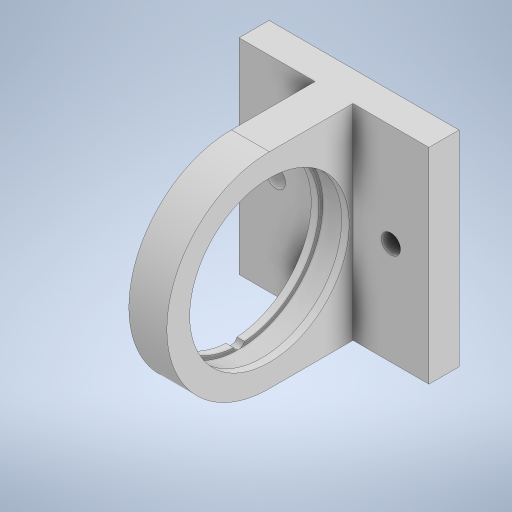
# Autodesk Inventor part: antenna_rad_outter
Saved by Autodesk Inventor 2024 (Build 280153000, 153)
## iProperties
Created: 2025-12-27
Part Number: antenna_rad_outter
Material: Generic
Document SubType Name: Modeling
Designer: schar
Density: 1 g/cm^3
Appearance: Default
Author: schar
Autodesk Inventor part; units mm, degrees
ref_plane "YZ Plane" through (0, 0, 0) normal (1, 0, 0) x (0, 1, 0)
ref_plane "XZ Plane" through (0, 0, 0) normal (0, 1, 0) x (-1, 0, 0)
sketch "Sketch15" plane through (0, 0, 0) normal (1, 0, 0) x (0, 1, 0)
  circle A0 centre (0, 0) radius 22
  circle A1 centre (0, 0) radius 27
  line L0 (27, 0) -> (27, -29.9149)
  line L1 (27, -29.9149) -> (-27, -29.9149)
  line L2 (-27, -29.9149) -> (-27, 0)
  dimension "d51" = 44
  dimension "d52" = 54
  constraints: 6 end point, 2 centre point, 2 coincident, 2 perpendicular, 2 point on circle, 1 vertical
  measures "d51" diameter of A0
  measures "d52" diameter of A1
extrude "Extrusion11" add sketch "Sketch15" along normal blind 10
sketch "Sketch16" plane through (10, 0, 0) normal (1, 0, 0) x (0, 0, -1)
  line L0 (29.9149, -27) -> (29.9149, 27) projected
  circle A0 centre (0, 0) radius 22 projected
  line L1 (29.9149, 27) -> (22, 27)
  line L2 (22, 27) -> (22, 0)
  line L3 (22, 0) -> (29.9149, 0)
  line L4 (29.9149, 0) -> (29.9149, 27)
  line L5 (0, -27) -> (29.9149, -27) projected
  line L6 (22, 0) -> (29.9149, 0)
  line L7 (29.9149, 0) -> (29.9149, -27)
  line L8 (29.9149, -27) -> (22, -27)
  line L9 (22, -27) -> (22, 0)
  constraints: 16 end point, 4 parallel, 2 horizontal, 2 perpendicular, 1 horizontal alignment, 1 other
extrude "Extrusion12" add sketch "Sketch16" along normal blind 20 contours L5 L9 L3 L0 | L3 L2 L1 L0
sketch "Sketch17" plane through (0, 0, 0) normal (-1, 0, 0) x (0, 0, 1)
  line L0 (-29.9149, -27) -> (-29.9149, 27) projected
  circle A0 centre (0, 0) radius 22 projected
  line L1 (-29.9149, 27) -> (-22, 27)
  line L2 (-22, 27) -> (-22, 0)
  line L3 (-22, 0) -> (-29.9149, 0)
  line L4 (-29.9149, 0) -> (-29.9149, 27)
  line L5 (0, -27) -> (-29.9149, -27) projected
  line L6 (-22, 0) -> (-29.9149, 0)
  line L7 (-29.9149, 0) -> (-29.9149, -27)
  line L8 (-29.9149, -27) -> (-22, -27)
  line L9 (-22, -27) -> (-22, 0)
  constraints: 16 end point, 4 parallel, 2 horizontal, 2 perpendicular, 1 horizontal alignment, 1 other
extrude "Extrusion13" add sketch "Sketch17" along normal blind 20 contours L0 L3 L9 L5 | L0 L1 L2 L3
ref_plane "Work Plane8" through (0, 0, 0) normal (0, -1, 0) x (1, 0, 0)
sketch "Sketch18" plane through (0, 0, 0) normal (0, -1, 0) x (1, 0, 0)
  line L0 (0, 0) -> (0, -22)
  line L1 (0, -22) -> (2, -22)
  line L2 (10, -22) -> (0, -22) projected
  line L3 (0, -22) -> (0, -21)
  line L4 (0, -21) -> (2, -21)
  line L5 (2, -22) -> (2, -21)
  line L6 (10, -22) -> (8, -22)
  line L7 (8, -22) -> (8, -21)
  line L8 (8, -21) -> (10, -21)
  line L9 (10, -21) -> (10, -22)
  line L10 (-30, 0) -> (40, 0) projected
  dimension "d59" = 2
  dimension "d60" = 1
  dimension "d61" = 2
  dimension "d62" = 1
  constraints: 18 end point, 5 perpendicular, 3 point on line
  measures "d59" distance of L0.end L1.end
  measures "d60" distance of L2.end L3.end
  measures "d61" distance of L2.start L6.end
  measures "d62" distance of L6.end L7.end
revolve "Revolution3" add sketch "Sketch18" angle 360 about axis through (-10, 0, 0) along (1, 0, 0)
sketch "Sketch19" plane through (10, -27, -22) normal (0, 0, 1) x (1, 0, 0)
  line L0 (20, 54) -> (20, 0) projected
  line L1 (20, 27) -> (10, 27)
  line L2 (-30.2682, 27) -> (-20.2682, 27)
  circle A0 centre (-20.2682, 27) radius 2.5
  circle A1 centre (10, 27) radius 2.5
  point P0 (-10, 27)
  dimension "d64" = 10
  dimension "d65" = 10
  dimension "d66" = 5
  dimension "d67" = 5
  constraints: 4 end point, 2 centre point, 2 coincident, 2 horizontal, 1 midpoint
  measures "d64" distance of L1.start L1.end
  measures "d65" distance of L2.start L2.end
  measures "d66" diameter of A0
  measures "d67" diameter of A1
extrude "Extrusion14" cut sketch "Sketch19" against normal blind 20
sketch "Sketch20" plane through (2, 0, 0) normal (1, 0, 0) x (0, 0, -1)
  circle A0 centre (0, 0) radius 22 projected
  line L0 (0, -22) -> (0, -20.5)
  circle A1 centre (0, -20.5) radius 1.5
  dimension "d71" = 1.5
  constraints: 2 end point, 2 vertical alignment, 1 coincident, 1 vertical, 3 other
  measures "d71" distance of L0.start L0.end
extrude "Extrusion15" cut sketch "Sketch20" against normal blind 20 contours A1
body "Solid3"
